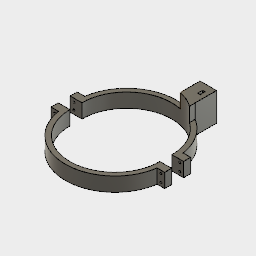
Scopeclamp v3 Motor v2 (Autodesk Fusion 360 design; units mm, degrees)
Autodesk Fusion 360 part; units mm, degrees
sketch "Sketch1" plane through (0, 0, 0) normal (0, 1, 0) x (1, 0, 0)
sketch "Sketch2" plane through (0, 0, 0) normal (0, 1, 0) x (1, 0, 0)
  circle A0 centre (0, 0) radius 105
  circle A1 centre (0, 0) radius 95
  line L0 (-120, 15) -> (-103.8566, 15)
  line L1 (-103.8566, 15) -> (-103.8566, -15.4532)
  line L2 (-103.8566, -15.4532) -> (-120, -15.4532)
  line L3 (-120, -15.4532) -> (-120, 15)
  line L4 (120, 15) -> (103.9026, 15)
  line L5 (103.9026, 15) -> (103.9026, -15)
  line L6 (103.9026, -15) -> (120, -15)
  line L7 (120, -15) -> (120, 15)
  line L8 (0, 105) -> (35, 105)
  line L9 (20, 135) -> (55, 135)
  line L10 (55, 135) -> (55, 89)
  line L11 (55, 89) -> (20, 89)
  line L12 (20, 89) -> (20, 135)
  dimension "d1" = 210
  dimension "d2" = 190
  dimension "d4" = 30
  measures "d1" diameter of A0
  measures "d2" diameter of A1
  measures "d4" distance of L4.start L6.end
extrude "Extrude1" add sketch "Sketch2" along normal blind 30 contours A0 L4 L5 L6 | A0 L4 L6 L7 | A0 A1 L0 L1 L4 L5 L6 L10 L11 L12 | A0 A1 L10 L11 L12 | A0 L9 L10 L12 | A0 L0 L2 L3 | A0 L0 L1 makes body 1
sketch "Sketch3" plane through (0, 30, 0) normal (0, 1, 0) x (-1, 0, 0)
  circle A0 centre (0, 0) radius 95
  line L0 (-20, -135) -> (-20, -103.0776)
  arc A1 (-20, -103.0776) -> (103.923, -15) centre (0, 0) ccw
  line L1 (103.923, -15) -> (120, -15)
  line L2 (120, -15) -> (120, 15.4532)
  line L3 (120, 15.4532) -> (103.8566, 15.4532)
  arc A2 (103.8566, 15.4532) -> (-103.923, 15) centre (0, 0) ccw
  line L4 (-103.923, 15) -> (-120, 15)
  line L5 (-120, 15) -> (-120, -15)
  line L6 (-120, -15) -> (-103.923, -15)
  arc A3 (-103.923, -15) -> (-55, -89.4427) centre (0, 0) ccw
  line L7 (-55, -89.4427) -> (-55, -135)
  line L8 (-55, -135) -> (-20, -135)
  line L9 (-55, -89.4427) -> (-55.1785, -77.3326)
  line L10 (-20, -103.0776) -> (-20.2896, -92.808)
extrude "Extrude2" add sketch "Sketch3" along normal blind 30 contours A0 L0 L7 L8 L9 L10 bodies 1
sketch "Sketch4" plane through (20, 0, 0) normal (-1, 0, 0) x (0, 0, 1)
  line L0 (-135, 0) -> (-103.0776, 0)
  line L1 (-103.0776, 0) -> (-103.0776, 30)
  line L2 (-103.0776, 30) -> (-103.0776, 60)
  line L3 (-103.0776, 60) -> (-135, 60)
  line L4 (-135, 60) -> (-135, 0)
  line L5 (-103.0776, 49.9607) -> (-123.0776, 49.9607)
  line L6 (-123.0776, 49.9607) -> (-123.0776, 9.9607)
  line L7 (-123.0776, 9.9607) -> (-103.0776, 9.9607)
  line L8 (-103.0776, 9.9607) -> (-103.0776, 49.9607)
  dimension "d9" = 20
  dimension "d10" = 40
  measures "d9" distance of L5.start L5.end
  measures "d10" distance of L5.start L7.end
extrude "Extrude3" cut sketch "Sketch4" against normal blind 30 contours L1 L2 L5 L6 L7 L8 bodies 1
sketch "Sketch5" plane through (0, 60, 0) normal (0, 1, 0) x (-1, 0, 0)
  line L0 (-55, -89.4427) -> (-55, -135)
  line L1 (-55, -135) -> (-20, -135)
  line L2 (-20, -135) -> (-20, -103.0776)
  line L3 (-20, -103.0776) -> (-20.2896, -92.808)
  arc A0 (-55.1785, -77.3326) -> (-20.2896, -92.808) centre (0, 0) ccw
  line L4 (-55.1785, -77.3326) -> (-55, -89.4427)
  line L5 (-45.0053, -120.2417) -> (-40.0053, -120.2417)
  line L6 (-40.0053, -120.2417) -> (-40.0053, -110.2417)
  line L7 (-40.0053, -110.2417) -> (-45.0053, -110.2417)
  line L8 (-45.0053, -110.2417) -> (-45.0053, -120.2417)
  dimension "d13" = 10
  dimension "d14" = 5
  measures "d13" distance of L5.start L7.end
  measures "d14" distance of L5.start L5.end
extrude "Extrude4" cut sketch "Sketch5" against normal blind 12 contours L5 L6 L7 L8 bodies 1
sketch "Sketch6" plane through (22.8885, 0, -0.6454) normal (-0.999603, 0, 0.028188) x (0.028188, 0, 0.999603)
  line L0 (-102.4729, 30) -> (-92.1992, 30)
  line L1 (-92.1992, 30) -> (-92.1992, 60)
  line L2 (-92.1992, 60) -> (-102.4729, 60)
  line L3 (-102.4729, 60) -> (-102.4729, 49.9607)
  line L4 (-102.4729, 49.9607) -> (-102.4729, 30)
split_face "SplitFace1" 1 faces at (-111.6661, 30, 0.3358) by plane through (0, 0, 0) normal (0, 0, 1) on bodies 1
hole "Hole1" at (111.8788, 23.9503, 15) direction (0, 0, -1) diameter 4 depth 40 tip angle 118 bodies 1
hole "Hole2" at (112.0186, 7.5747, 15) direction (0, 0, -1) diameter 4 depth 40 tip angle 118 bodies 1
hole "Hole3" at (-111.8476, 22.6099, -15) direction (0, 0, 1) diameter 4 depth 40 tip angle 118 bodies 1
hole "Hole4" at (-112.145, 8.1428, -15) direction (0, 0, 1) diameter 4 depth 40 tip angle 118 bodies 1
split "Split1" by plane through (0, 0, 0) normal (0, 0, 1) bodies 1 makes body 2 at (72.5134, 20, 75.9395)
copy_body "CutPasteBodies1" bodies 2 removing the originals makes body 3
copy_body "CutPasteBodies2" bodies 3 removing the originals makes body 4
move_body "Move1" bodies 4 to x (1, 0, 0) y (0, 1, 0) z (0, 0, 1) at (0, 0, 25)
